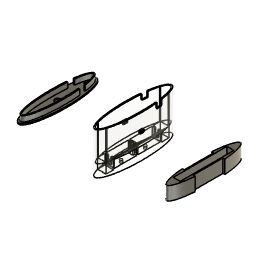
Boby_and_BatteryHolder_OutwardMotors (Autodesk Fusion 360 design; units mm, degrees)
Autodesk Fusion 360 part; units mm, degrees
sketch "Sketch1" plane through (0, 0, 0) normal (0, 0, 1) x (1, 0, 0)
  ellipse E0 centre (0, 0) end of major axis (0, -27.7) minor radius 5.65
  line L0 (0, 27.7) -> (0, -27.7) construction
  line L1 (-5.65, 0) -> (5.65, 0) construction
  ellipse E1 centre (0, 0) end of major axis (0, -28.7) minor radius 6.65
  line L2 (0, 28.7) -> (0, -28.7) construction
  line L3 (-6.65, 0) -> (6.65, 0) construction
  line L4 (3.05, -1.8) -> (3.05, -17.2)
  line L5 (3.05, -17.2) -> (-3.05, -17.2)
  line L6 (-3.05, -17.2) -> (-3.05, -1.8)
  line L7 (-3.05, -1.8) -> (3.05, -1.8)
  line L8 (-3.2, -17.9) -> (3.2, -17.9)
  line L9 (3.2, -17.9) -> (3.2, -23.4)
  line L10 (3.2, -23.4) -> (-3.2, -23.4)
  line L11 (-3.2, -23.4) -> (-3.2, -17.9)
  line L12 (-1.2, -17.2) -> (-1.2, -17.9)
  line L13 (1.2, -17.2) -> (1.2, -17.9)
  line L14 (-5.65, 0) -> (5.65, 0)
  line L15 (-3.05, 1.8) -> (3.05, 1.8)
  line L16 (-3.05, 17.2) -> (-3.05, 1.8)
  line L17 (3.05, 1.8) -> (3.05, 17.2)
  line L18 (3.05, 17.2) -> (-3.05, 17.2)
  line L19 (-1.2, 17.2) -> (-1.2, 17.9)
  line L20 (1.2, 17.2) -> (1.2, 17.9)
  line L21 (-3.2, 17.9) -> (3.2, 17.9)
  line L22 (-3.2, 23.4) -> (-3.2, 17.9)
  line L23 (3.2, 23.4) -> (-3.2, 23.4)
  line L24 (3.2, 17.9) -> (3.2, 23.4)
  line L25 (1.5209, 1.8) -> (1.5209, 0.5)
  line L26 (1.5209, 0.5) -> (3.05, 0.5)
  line L27 (3.05, 0.5) -> (3.05, 1.8)
  line L28 (-3.05, 1.8) -> (-3.05, 0.5)
  line L29 (-3.05, 0.5) -> (-1.5, 0.5)
  line L30 (-1.5, 0.5) -> (-1.5, 1.8)
  line L31 (-3.05, -1.8) -> (-3.05, -0.5)
  line L32 (-3.05, -0.5) -> (-1.5, -0.5)
  line L33 (-1.5, -0.5) -> (-1.5, -1.8)
  line L34 (3.05, -1.8) -> (3.05, -0.5)
  line L35 (3.05, -0.5) -> (1.5, -0.5)
  line L36 (1.5, -0.5) -> (1.5, -1.8)
  ellipse E2 centre (49.4, 3) end of major axis (49.4, -24.5) minor radius 5.25
  line L37 (49.4, 30.5) -> (49.4, -24.5) construction
  line L38 (44.15, 3) -> (54.65, 3) construction
  line L39 (46.8, 23) -> (52, 23)
  line L40 (52, 23) -> (52, -17)
  line L41 (52, -17) -> (46.8, -17)
  line L42 (46.8, -17) -> (46.8, 23)
  circle A0 centre (0, 9) radius 1
  circle A1 centre (0, -9) radius 1
  circle A2 centre (0, -9) radius 1
  line L43 (-3.05, -0.5) -> (-1.5, -0.5)
  line L44 (3.05, -17.2) -> (-3.05, -17.2)
  line L45 (-1.5, 0.5) -> (-1.5, 1.8)
  line L46 (3.2, -23.4) -> (-3.2, -23.4)
  line L47 (1.5209, 0.5) -> (3.05, 0.5)
  line L48 (-1.5, -0.5) -> (-1.5, -1.8)
  line L49 (-3.05, -1.8) -> (3.05, -1.8)
  line L50 (3.05, 0.5) -> (3.05, 1.8)
  line L51 (3.05, -1.8) -> (3.05, -17.2)
  line L52 (-1.2, -17.2) -> (-1.2, -17.9)
  line L53 (-3.2, -23.4) -> (-3.2, -17.9)
  line L54 (-5.65, 0) -> (5.65, 0)
  line L55 (-3.2, 17.9) -> (3.2, 17.9)
  line L56 (3.2, 17.9) -> (3.2, 23.4)
  line L57 (-3.2, 23.4) -> (-3.2, 17.9)
  line L58 (-3.05, 1.8) -> (-3.05, 0.5)
  circle A3 centre (0, 9) radius 1
  line L59 (1.2, -17.2) -> (1.2, -17.9)
  line L60 (-3.2, -17.9) -> (3.2, -17.9)
  line L61 (-3.05, 17.2) -> (-3.05, 1.8)
  line L62 (3.2, 23.4) -> (-3.2, 23.4)
  line L63 (3.05, -0.5) -> (1.5, -0.5)
  line L64 (1.5, -0.5) -> (1.5, -1.8)
  line L65 (-3.05, 1.8) -> (3.05, 1.8)
  line L66 (1.2, 17.2) -> (1.2, 17.9)
  line L67 (3.05, 1.8) -> (3.05, 17.2)
  line L68 (-3.05, 0.5) -> (-1.5, 0.5)
  line L69 (-3.05, -1.8) -> (-3.05, -0.5)
  line L70 (-1.2, 17.2) -> (-1.2, 17.9)
  line L71 (3.05, -1.8) -> (3.05, -0.5)
  line L72 (-3.05, -17.2) -> (-3.05, -1.8)
  line L73 (3.2, -17.9) -> (3.2, -23.4)
  line L74 (1.5209, 1.8) -> (1.5209, 0.5)
  ellipse E3 centre (0, 0) end of major axis (0, -27.7) minor radius 5.65
  line L75 (0, 27.7) -> (0, -27.7) construction
  line L76 (-5.65, 0) -> (5.65, 0) construction
  ellipse E4 centre (0, 0) end of major axis (0, -28.7) minor radius 6.65
  line L77 (0, 28.7) -> (0, -28.7) construction
  line L78 (-6.65, 0) -> (6.65, 0) construction
  line L79 (3.05, 17.2) -> (-3.05, 17.2)
  line L80 (54.2121, -7.9949) -> (52.8, -7.9949)
  line L81 (52.8, -7.9949) -> (52.8, 13.9949)
  line L82 (52.8, 13.9949) -> (54.2121, 13.9949)
  line L83 (49.4, 8.1519) -> (49.4, -5) construction
  line L84 (46, 13.9949) -> (44.5879, 13.9949)
  line L85 (46, -7.9949) -> (46, 13.9949)
  line L86 (44.5879, -7.9949) -> (46, -7.9949)
  circle A4 centre (49.4, 3) radius 1.5
  point P0 (54.65, 3)
  dimension "d86" = 55.4
  dimension "d87" = 11.3
  dimension "d88" = 57.4
  dimension "d89" = 13.3
  dimension "d90" = 15.4
  dimension "d91" = 3.05
  dimension "d92" = 3.05
  dimension "d97" = 5.5
  dimension "d98" = 6.4
  dimension "d99" = 0.7
  dimension "d100" = 10.5
  dimension "d101" = 1.2
  dimension "d102" = 1.2
  dimension "d103" = 55
  dimension "d104" = 10.5
  dimension "d105" = 5.2
  dimension "d106" = 2.6
  dimension "d107" = 40
  dimension "d108" = 20
  dimension "d111" = 2
  dimension "d112" = 2
  dimension "d136" = 55.4
  dimension "d137" = 11.3
  dimension "d138" = 57.4
  dimension "d139" = 13.3
  dimension "d140" = 15.4
  dimension "d141" = 3.05
  dimension "d142" = 3.05
  dimension "d143" = 5.5
  dimension "d144" = 6.4
  dimension "d145" = 0.7
  dimension "d146" = 10.5
  dimension "d147" = 1.2
  dimension "d148" = 1.2
  dimension "d149" = 2
  dimension "d150" = 2
  dimension "d230" = 3
  constraint coincident E0 L0.start
  constraint coincident E0 L0.end
  constraint coincident E0 L1.start
  constraint coincident E0 L1.end
  constraint coincident E0.centre E1.centre
  constraint vertical L0
  constraint coincident E1 L2.start
  constraint coincident E1 L2.end
  constraint coincident E1 L3.start
  constraint coincident E1 L3.end
  constraint perpendicular L1 L2
  constraint perpendicular L1 L4
  constraint perpendicular L0 L5
  constraint perpendicular L4 L7
  constraint horizontal L8
  constraint vertical L9
  constraint horizontal L10
  constraint vertical L11
  constraint coincident L5 L12.start
  constraint coincident L8 L12.end
  constraint perpendicular L8 L12
  constraint coincident L5 L13.start
  constraint coincident L8 L13.end
  constraint perpendicular L8 L13
  constraint coincident L1.start L14.start
  constraint coincident L1.end L14.end
  constraint symmetric L4.end L14 L17.end
  constraint symmetric L5.end L14 L16.start
  constraint symmetric L6.end L14 L15.start
  constraint symmetric L4.start L14 L15.end
  constraint symmetric L8.start L14 L21.start
  constraint symmetric L8.end L14 L21.end
  constraint symmetric L9.end L14 L23.start
  constraint symmetric L10.end L14 L22.start
  constraint symmetric L12.start L14 L19.start
  constraint symmetric L12.end L14 L19.end
  constraint symmetric L13.start L14 L20.start
  constraint symmetric L13.end L14 L20.end
  constraint coincident L15 L25.start
  constraint perpendicular L15 L25
  constraint perpendicular L17 L26
  constraint perpendicular L15 L27
  constraint perpendicular L15 L28
  constraint perpendicular L16 L29
  constraint coincident L15 L30.end
  constraint perpendicular L15 L30
  constraint perpendicular L7 L31
  constraint perpendicular L6 L32
  constraint coincident L7 L33.end
  constraint perpendicular L7 L33
  constraint perpendicular L7 L34
  constraint perpendicular L4 L35
  constraint coincident L7 L36.end
  constraint perpendicular L7 L36
  constraint coincident E2 L37.start
  constraint coincident E2 L37.end
  constraint coincident E2 L38.start
  constraint coincident E2 P0
  constraint vertical L37
  constraint perpendicular L37 L39
  constraint perpendicular L39 L40
  constraint perpendicular L37 L41
  constraint perpendicular L39 L42
  constraint coincident L2 A0.centre
  constraint coincident L0 A1.centre
  constraint coincident L0.start E3
  constraint coincident L0.end E3
  constraint coincident L1.start E3
  constraint coincident L1.end E3
  constraint vertical L75
  constraint coincident L2.start E4
  constraint coincident L2.end E4
  constraint coincident L3.start E4
  constraint coincident L3.end E4
  constraint perpendicular L76 L77
  constraint perpendicular L51 L76
  constraint perpendicular L44 L75
  constraint perpendicular L49 L51
  constraint horizontal L60
  constraint vertical L73
  constraint horizontal L46
  constraint vertical L53
  constraint coincident L12.start L44
  constraint coincident L12.end L60
  constraint perpendicular L52 L60
  constraint coincident L13.start L44
  constraint coincident L13.end L60
  constraint perpendicular L59 L60
  constraint symmetric L17.end L4.end L54
  constraint symmetric L5.end L16.start L54
  constraint symmetric L15.start L6.end L54
  constraint symmetric L4.start L15.end L54
  constraint symmetric L21.start L8.start L54
  constraint symmetric L21.end L8.end L54
  constraint symmetric L23.start L9.end L54
  constraint symmetric L22.start L10.end L54
  constraint symmetric L19.start L12.start L54
  constraint symmetric L19.end L12.end L54
  constraint symmetric L13.start L20.start L54
  constraint symmetric L20.end L13.end L54
  constraint coincident L25.start L65
  constraint perpendicular L65 L74
  constraint perpendicular L47 L67
  constraint perpendicular L50 L65
  constraint perpendicular L58 L65
  constraint perpendicular L61 L68
  constraint coincident L30.end L65
  constraint perpendicular L45 L65
  constraint perpendicular L49 L69
  constraint perpendicular L43 L72
  constraint coincident L33.end L49
  constraint perpendicular L48 L49
  constraint perpendicular L49 L71
  constraint perpendicular L51 L63
  constraint coincident L36.end L49
  constraint perpendicular L49 L64
  constraint coincident A0.centre L77
  constraint coincident A1.centre L75
  constraint horizontal L80
  constraint perpendicular L80 L81
  constraint parallel L80 L82
  constraint coincident P0 L38.end
  constraint coincident E2 L82.end
  constraint coincident E2 L80.start
  constraint coincident L37 L83.start
  constraint coincident L37 L83.end
  constraint perpendicular L38 L83
  constraint symmetric L80.end L83 L85.start
  constraint symmetric L81.end L83 L84.start
  constraint symmetric L82.end L83 L84.end
  constraint symmetric L80.start L83 L86.start
  constraint concentric E2 A4
  measures "d86" distance of E0
  measures "d88" distance of E1
  measures "d90" distance of L5 L7
  measures "d91" distance of L0 L4
  measures "d92" distance of L2 L6
  measures "d97" distance of L8 L10
  measures "d98" distance of L9 L11
  measures "d99" distance of L5 L8
  measures "d100" distance of L0.end L5
  measures "d101" distance of L2 L13
  measures "d102" distance of L2 L12
  measures "d103" distance of E2
  measures "d105" distance of L40 L42
  measures "d106" distance of L37 L40
  measures "d107" distance of L39 L41
  measures "d108" distance of L38 L41
  measures "d111" diameter of A0
  measures "d112" diameter of A1
  measures "d136" distance of E3
  measures "d138" distance of E4
  measures "d140" distance of L44 L49
  measures "d141" distance of L51 L75
  measures "d142" distance of L72 L77
  measures "d143" distance of L46 L60
  measures "d144" distance of L53 L73
  measures "d145" distance of L44 L60
  measures "d146" distance of L0.end L44
  measures "d147" distance of L59 L77
  measures "d148" distance of L52 L77
  measures "d149" diameter of A3
  measures "d150" diameter of A2
  measures "d230" diameter of A4
extrude "Extrude27" add sketch "Sketch1" against normal blind 8.5 contours E0 L10 L46 E3 | E0 L8 L9 L10 L11 L46 L53 L60 L73 E3 | E0 L9 L10 L46 L73 E3 | E0 L10 L11 L46 L53 E3 | E0 L4 L5 L6 L7 L8 L9 L11 L12 L13 L14 L31 L32 L33 L34 L35 L36 L43 L44 L48 L49 L51 L52 L53 L54 L59 L60 L63 L64 L69 L71 L72 L73 E3 | E0 L14 L15 L16 L17 L18 L19 L20 L21 L22 L24 L25 L26 L27 L28 L29 L30 L45 L47 L50 L54 L55 L56 L57 L58 L61 L65 L66 L67 L68 L70 L74 E3 L79 | E0 L21 L22 L23 L24 L55 L56 L57 L62 E3 | E0 L23 L24 L56 L62 E3 | L5 L8 L12 L13 L44 L52 L59 L60 | E0 L22 L23 L57 L62 E3 | E0 L23 L62 E3 | L4 L5 L6 L7 L44 L49 L51 L72 | L18 L19 L20 L21 L55 L66 L70 L79 | L15 L16 L17 L18 L61 L65 L67 L79 | L7 L34 L35 L36 L49 L63 L64 L71 | L7 L31 L32 L33 L43 L48 L49 L69 | L15 L25 L26 L27 L47 L50 L65 L74 | L15 L28 L29 L30 L45 L58 L65 L68 | E1 E4 | A0 A3 | A1 A2 makes body 1
extrude "Extrude28" cut sketch "Sketch1" against normal blind 10 contours A0 A3 | A1 A2 bodies 1
extrude "Extrude29" cut sketch "Sketch1" against normal blind 7 contours L4 L5 L6 L7 L44 L49 L51 L72 | L15 L16 L17 L18 L61 L65 L67 L79 | L7 L34 L35 L36 L49 L63 L64 L71 | L7 L31 L32 L33 L43 L48 L49 L69 | L15 L25 L26 L27 L47 L50 L65 L74 | L15 L28 L29 L30 L45 L58 L65 L68 bodies 1
extrude "Extrude30" cut sketch "Sketch1" against normal blind 7.5 contours E0 L8 L9 L10 L11 L46 L53 L60 L73 E3 bodies 1
extrude "Extrude31" cut sketch "Sketch1" against normal blind 7.5 contours E0 L21 L22 L23 L24 L55 L56 L57 L62 E3 bodies 1
extrude "Extrude32" cut sketch "Sketch1" against normal blind 5.5 contours L5 L8 L12 L13 L44 L52 L59 L60 | L18 L19 L20 L21 L55 L66 L70 L79 bodies 1
extrude "Extrude33" cut sketch "Sketch1" against normal blind 7.5 contours E0 L9 L10 L46 L73 E3 | E0 L10 L11 L46 L53 E3 | E0 L23 L24 L56 L62 E3 | E0 L22 L23 L57 L62 E3 bodies 1
extrude "Extrude35" add sketch "Sketch1" along normal blind 13.5 contours E1 E4 bodies 1
ref_plane "WorkPlane1" through (0, 0, 11) normal (0, 0, 1) x (1, 0, 0)
sketch "Sketch2" plane through (0, 0, 11) normal (0, 0, 1) x (1, 0, 0)
  line L0 (-8, 1.5) -> (8, 1.5)
  line L1 (8, 1.5) -> (8, -1.5)
  line L2 (8, -1.5) -> (-8, -1.5)
  line L3 (-8, -1.5) -> (-8, 1.5)
  constraint horizontal L0
  constraint perpendicular L0 L1
  constraint perpendicular L1 L2
  constraint perpendicular L0 L3
extrude "Extrude37" cut sketch "Sketch2" against normal blind 2 bodies 1
extrude "Extrude38" add 1 faces at (5.7335, 6.3692, 13.5) along direction (0, 0, 1) blind 9 on bodies 1 bodies 1
sketch "Sketch3" plane through (0, 0, 0) normal (0, 0, 1) x (1, 0, 0)
  ellipse E0 centre (-55, -1.35) end of major axis (-55, -28.825) minor radius 5.425
  line L0 (-55, 26.125) -> (-55, -28.825) construction
  ellipse E1 centre (-55, -1.35) end of major axis (-55, -30.45) minor radius 7.05
  line L1 (-55, 27.75) -> (-55, -30.45) construction
  ellipse E2 centre (-55, -1.35) end of major axis (-55, -27.825) minor radius 4.425
  line L2 (-55, 25.125) -> (-55, -27.825) construction
  line L3 (-59.425, -1.35) -> (-50.575, -1.35) construction
  line L4 (-50.5, 4.25) -> (-59.5, 4.25)
  line L5 (-59.5, 4.25) -> (-59.5, 19.75)
  line L6 (-59.5, 19.75) -> (-50.5, 19.75)
  line L7 (-50.5, 19.75) -> (-50.5, 4.25)
  line L8 (-50.5, 4.25) -> (-59.5, 19.75) construction
  line L9 (-59.5, 4.25) -> (-50.5, 19.75) construction
  line L10 (-59.396, 14.75) -> (-50.604, 14.75)
  line L11 (-59.9178, 10.25) -> (-50.0822, 10.25)
  circle A0 centre (-55, -1.35) radius 2
  circle A1 centre (-55, 21.025) radius 2
  circle A2 centre (-55, -23.725) radius 2
  point P0 (-55, 12)
  dimension "d151" = 54.95
  dimension "d152" = 10.85
  dimension "d153" = 58.2
  dimension "d154" = 14.1
  dimension "d166" = 52.95
  dimension "d167" = 8.85
  dimension "d170" = 9
  dimension "d171" = 15.5
  dimension "d172" = 8
  dimension "d191" = 5
  dimension "d192" = 6
  dimension "d209" = 4
  dimension "d210" = 4
  dimension "d211" = 4.1
  dimension "d212" = 4
  dimension "d213" = 4.1
  constraint coincident L0.start E0
  constraint coincident L0.end E0
  constraint vertical L0
  constraint coincident L1.start E1
  constraint coincident L1.end E1
  constraint coincident E0.centre E1.centre
  constraint coincident E2 L2.start
  constraint coincident E2 L2.end
  constraint coincident E2 L3.start
  constraint coincident E2 L3.end
  constraint concentric E0 E2
  constraint parallel L1 L2
  constraint horizontal L4
  constraint perpendicular L4 L5
  constraint parallel L4 L6
  constraint parallel L5 L7
  constraint coincident L8 P0
  constraint coincident L9 P0
  constraint coincident L0 P0
  constraint coincident L1 P0
  constraint coincident E0 L10.start
  constraint coincident E0 L10.end
  constraint horizontal L10
  constraint coincident E0 L11.start
  constraint coincident E0 L11.end
  constraint perpendicular L7 L11
  constraint concentric E2 A0
  constraint coincident L0 A1.centre
  constraint coincident L0 A2.centre
  measures "d151" distance of E0
  measures "d153" distance of E1
  measures "d166" distance of E2
  measures "d170" distance of L5.end L6.end
  measures "d171" distance of L4.end L5.end
  measures "d172" distance of L1.start L6
  measures "d191" distance of L6 L10
  measures "d192" distance of L4 L11
  measures "d209" diameter of A0
  measures "d210" diameter of A1
  measures "d211" distance of L2.start A1.centre
  measures "d212" diameter of A2
  measures "d213" distance of L2.end A2.centre
extrude "Extrude47" add sketch "Sketch3" against normal blind 1 separate body contours E0 E2 L4 L5 L7 L11 | E0 L7 L11 | E0 L5 L11 | E0 E2 L7 L10 L11 | E0 L6 L7 | E2 L4 L7 L11 | E0 L5 L6 | E0 E2 L5 L10 L11 | E2 L4 L5 L11 | E0 E2 L6 L10 | E2 L10 L11 | E0 E2 L6 L10 | E0 E2 L6 | E2 L4 | E2 L6 A1 | L6 A1 | E1 | A0 | A2 picked at (-55.0338, 20.8408) makes body 2
extrude "Extrude48" add sketch "Sketch3" along normal blind 4 contours E0 E2 L4 L5 L7 L11 | E2 L4 L7 L11 | E2 L4 L5 L11 | E0 E2 L6 L10 | E0 E2 L6 L10 | E0 E2 L6 bodies 2
sketch "Sketch4" plane through (0, 0, 22.5) normal (0, 0, 1) x (-1, 0, 0)
  line L0 (-3.2, 22.829) -> (-3.2, 23.4)
  line L1 (-3.2, 23.4) -> (-3.0235, 23.4)
  ellipse E0 centre (0, 0) end of major axis (0, 27.7) minor radius 5.65 (3.0235, 23.4) -> (-3.0235, 23.4) ccw
  line L2 (3.0235, 23.4) -> (3.2, 23.4)
  line L3 (3.2, 23.4) -> (3.2, 22.829)
  ellipse E1 centre (0, 0) end of major axis (0, 27.7) minor radius 5.65 (3.2, -22.829) -> (3.2, 22.829) ccw
  line L4 (3.2, -22.829) -> (3.2, -23.4)
  line L5 (3.2, -23.4) -> (3.0235, -23.4)
  ellipse E2 centre (0, 0) end of major axis (0, 27.7) minor radius 5.65 (-3.0235, -23.4) -> (3.0235, -23.4) ccw
  line L6 (-3.0235, -23.4) -> (-3.2, -23.4)
  line L7 (-3.2, -23.4) -> (-3.2, -22.829)
  ellipse E3 centre (0, 0) end of major axis (0, 27.7) minor radius 5.65 (-3.2, 22.829) -> (-3.2, -22.829) ccw
  ellipse E4 centre (0, 0) end of major axis (0, 28.7) minor radius 6.65
  line L8 (-6.655, -11.7) -> (6.7101, -11.7)
  line L9 (6.7101, -11.7) -> (6.7101, -15.7)
  line L10 (6.7101, -15.7) -> (-6.655, -15.7)
  line L11 (-6.655, -15.7) -> (-6.655, -11.7)
  line L12 (-6.655, -11.7) -> (6.7101, -15.7) construction
  line L13 (6.7101, -11.7) -> (-6.655, -15.7) construction
  point P0 (0, -28.7)
  point P1 (0.0276, -13.7)
  dimension "d199" = 4
  dimension "d200" = 13
  constraint horizontal L8
  constraint perpendicular L8 L9
  constraint parallel L8 L10
  constraint parallel L9 L11
  constraint coincident L12 P1
  constraint coincident L13 P1
  measures "d199" distance of L8.end L9.end
  measures "d200" distance of P0 L10
extrude "Extrude49" cut sketch "Sketch4" against normal blind 4 contours E1 E3 L8 L10 | E3 E4 L8 L10 | E1 E4 L8 L10 bodies 1
extrude "Extrude50" add sketch "Sketch3" against normal blind 1.5 contours E2 L4 L11 | E2 L6 L10 A1 | L6 A1 picked at (-55.446, 19.6795) bodies 2
extrude "Extrude51" cut sketch "Sketch3" against normal blind 2 contours L6 A1 | L6 A1 | A0 | A2 bodies 2
chamfer "Chamfer3" distance 1.2 distance2 2.5 1 edges at (0, -1.8, 0) measured on face at (-4.6115, -4.0202, 0) on bodies 1
chamfer "Chamfer4" distance 1.2 distance2 2.5 1 edges at (0.0104, 1.8, 0) measured on face at (-4.6115, -4.0202, 0) on bodies 1
extrude "Extrude53" add sketch "Sketch1" against normal blind 1 separate body contours E2 L80 L81 L82 L84 L85 L86 | L39 L40 L41 L42 | A4 makes body 3
extrude "Extrude54" add sketch "Sketch1" along normal blind 9 contours E2 L80 L81 L82 L84 L85 L86 bodies 3
extrude "Extrude55" cut sketch "Sketch1" against normal blind 2 contours A4 bodies 3
equation "d88 = d136 + 2 mm"
equation "d89 = d137 + 2 mm"
equation "d103 = d86 - 0.4 mm"
equation "d104 = d87 - 0.8 mm"
equation "d136 = d86"
equation "d137 = d87"
equation "d138 = d88"
equation "d139 = d89"
